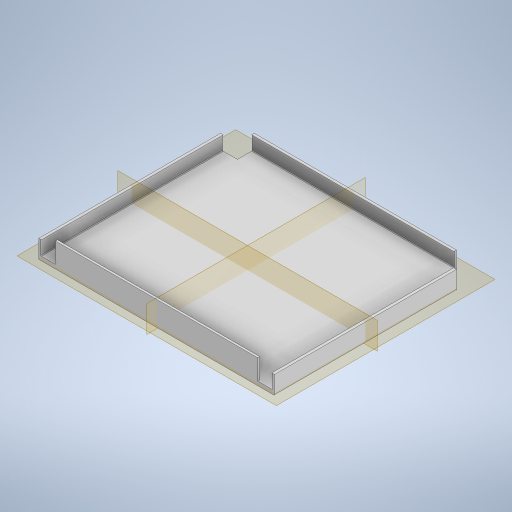
# Autodesk Inventor part: deckel
Saved by Autodesk Inventor 2023 (Build 270158000, 158)
## iProperties
Created: 2025-07-28
Part Number: deckel
Material: Generisch
Document SubType Name: Modeling
Designer: johan
Density: 1 g/cm^3
Appearance: Vorgabe
Author: johan
Autodesk Inventor part; units mm, degrees
sketch "Skizze1" plane through (0, 0, 0) normal (0, 1, 0) x (-1, 0, 0)
  line L0 (75, 67.5) -> (-75, 67.5)
  line L1 (-75, 67.5) -> (-75, -67.5)
  line L2 (-75, -67.5) -> (75, -67.5)
  line L3 (75, -67.5) -> (75, 67.5)
  line L4 (75, 67.5) -> (-75, -67.5) construction
  line L5 (-75, 67.5) -> (75, -67.5) construction
  point P0 (0, 0)
  dimension "d0" = 150
  dimension "d1" = 135
  constraints: 12 end point, 2 midpoint, 2 parallel, 1 horizontal, 1 perpendicular
  measures "d0" distance of L2.end L1.end
  measures "d1" distance of L1.end L0.end
extrude "Extrusion1" add sketch "Skizze1" along normal mid plane 3
sketch "Skizze2" plane through (0, 1.5, 0) normal (0, 1, 0) x (1, 0, 0)
  line L0 (-75, 67.5) -> (-75, -67.5) projected
  line L1 (75, -67.5) -> (75, 67.5) projected
  line L2 (-75, -67.5) -> (75, -67.5)
  line L3 (75, -67.5) -> (75, -66)
  line L4 (75, -66) -> (-75, -66)
  line L5 (-75, -66) -> (-75, -67.5)
  point P0 (0, 0)
  dimension "d4" = 135
  dimension "d5" = 1.5
  constraints: 8 end point, 2 parallel, 1 horizontal, 1 perpendicular, 1 point on line
  measures "d4" distance of L0.start L0.end
  measures "d5" distance of L3.end L2.end
extrude "Extrusion2" add sketch "Skizze2" along normal blind 15
sketch "Skizze3" plane through (0, 0, 0) normal (1, 0, 0) x (0, 1, 0)
  line L0 (1.5, -67.5) -> (1.5, 66) projected
  line L1 (1.5, -67.5) -> (-1.5, -67.5)
  line L2 (-1.5, -67.5) -> (-1.5, -77.5)
  line L3 (-1.5, -77.5) -> (1.5, -77.5)
  line L4 (1.5, -77.5) -> (1.5, -67.5)
  line L5 (2, -78.5) -> (11.5, -78.5)
  line L6 (1.5, -77.5) -> (1.5, -78)
  line L7 (-1.5, -77.5) -> (-1.5, -79.5)
  arc A0 (1.5, -78) -> (2, -78.5) centre (2, -78) ccw
  line L8 (12, -78.5) -> (12, -80)
  line L9 (12, -80) -> (-1, -80)
  arc A1 (-1.5, -79.5) -> (-1, -80) centre (-1, -79.5) ccw
  line L10 (12, -78) -> (12, -78)
  arc A2 (11.5, -78.5) -> (12, -78) centre (11.5, -78) ccw
  line L11 (12, -78.5) -> (12, -78)
  point P0 (0, 0)
  dimension "d8" = 10
  dimension "d16" = 1.5
  dimension "d17" = 0.5
  dimension "d19" = 10
  dimension "d20" = 0.5
  constraints: 22 end point, 7 tangent, 6 point on circle, 4 vertical, 3 centre point, 2 horizontal, 2 parallel, 2 perpendicular, 2 point on line
  measures "d8" distance of L2.end L1.end
  measures "d16" distance of L8.start L8.end
  measures "d17" radius of A1
  measures "d19" distance of L5.start L8.start
  measures "d20" distance of L8.start L10.end
extrude "Extrusion3" add sketch "Skizze3" along normal mid plane 150
sketch "Skizze5" plane through (0, 0, 0) normal (0, 0, 1) x (1, 0, 0)
  line L0 (75, 16.5) -> (75, -1.5) projected
  line L1 (75, -1.5) -> (87, -1.5)
  line L2 (87.5, -1) -> (87.5, 12)
  line L3 (85.5, 12) -> (85.5, 12)
  line L4 (86, 11.5) -> (86, 2)
  arc A0 (86, 11.5) -> (85.5, 12) centre (85.5, 11.5) ccw
  line L5 (85.5, 12) -> (87.5, 12)
  line L6 (75, 1.5) -> (85.5, 1.5)
  line L7 (75, -1.5) -> (-75, -1.5) projected
  line L8 (75, -1.5) -> (75, 1.5)
  arc A1 (85.5, 1.5) -> (86, 2) centre (85.5, 2) ccw
  arc A2 (87, -1.5) -> (87.5, -1) centre (87, -1) ccw
  line L9 (-75, -1.5) -> (-75, 16.5) projected
  line L10 (-75, -1.5) -> (-87, -1.5)
  line L11 (-87.5, -1) -> (-87.5, 12)
  line L12 (-85.5, 12) -> (-85.5, 12)
  line L13 (-86, 11.5) -> (-86, 2)
  line L14 (-85.5, 1.5) -> (-75, 1.5)
  line L15 (-75, 1.5) -> (-75, -1.5)
  arc A3 (-85.5, 12) -> (-86, 11.5) centre (-85.5, 11.5) ccw
  line L16 (-87.5, 12) -> (-85.5, 12)
  arc A4 (-86, 2) -> (-85.5, 1.5) centre (-85.5, 2) ccw
  arc A5 (-87.5, -1) -> (-87, -1.5) centre (-87, -1) ccw
  point P0 (0, 0)
  point P1 (87.5, -1.5)
  point P2 (-87.5, -1.5)
  point P3 (-86, 12)
  point P4 (-86, 1.5)
  dimension "d39" = 13.5
  dimension "d42" = 0.5
  dimension "d43" = 0.5
  dimension "d44" = 12.5
  dimension "d45" = 1.5
  dimension "d46" = 2
  dimension "d48" = 10.5
  dimension "d49" = 12.5
  dimension "d50" = 13.5
  dimension "d51" = 2
  dimension "d52" = 10.5
  dimension "d53" = 0.5
  dimension "d54" = 0.5
  constraints: 28 end point, 14 tangent, 12 point on circle, 12 point on line, 6 centre point, 6 horizontal, 3 perpendicular, 3 vertical, 2 equal radius, 1 collinear
  measures "d39" distance of point (87.5, -1.5) L2.end
  measures "d42" radius of A0
  measures "d43" radius of A1
  measures "d44" distance between parallel lines of L2 L8
  measures "d45" distance between parallel lines of L2 L4
  measures "d46" distance of L2.end L3.start
  measures "d48" distance from line of L6.end L8
  measures "d49" distance of L7.end point (-87.5, -1.5)
  measures "d50" distance of point (-87.5, -1.5) L11.end
  measures "d51" distance of L11.end L12.end
  measures "d52" distance of point (-86, 12) point (-86, 1.5)
  measures "d53" radius of A3
  measures "d54" radius of A4
extrude "Extrusion4" add sketch "Skizze5" along normal mid plane 135
